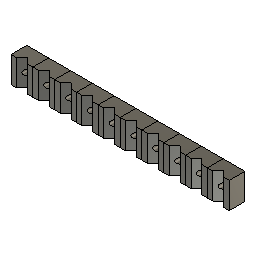
model (Autodesk Fusion 360 design; units mm, degrees)
Autodesk Fusion 360 part; units mm, degrees
sketch "profile" plane through (0, 0, 0) normal (0, 0, 1) x (1, 0, 0) in component "rail"
  line L0 (0, 0) -> (25, 0)
  line L1 (25, 0) -> (25, -18)
  line L2 (0, -18) -> (0, 0)
  line L3 (6.25, -18) -> (12.5, -11.75)
  line L4 (12.5, -11.75) -> (18.75, -18)
  line L5 (25, -18) -> (18.75, -18)
  line L6 (6.25, -18) -> (0, -18)
  line L7 (9.325, -14.925) -> (9.325, -8.575)
  line L8 (9.325, -8.575) -> (15.675, -8.575)
  line L9 (15.675, -8.575) -> (15.675, -14.925)
  line L10 (12.5, -11.75) -> (12.5, -8.575) construction
  line L11 (6.25, -18) -> (12.5, -18) construction
  line L12 (12.5, -18) -> (18.75, -18) construction
  dimension "d4" = 25
  dimension "d6" = 3.175
  dimension "d8" = 18
  dimension "d9" = 6.35
  dimension "d10" = 11.75
  constraint horizontal L0
  constraint vertical L1
  constraint horizontal L5
  constraint vertical L2
  constraint coincident L0.start L2.end
  constraint coincident L3.start L5
  constraint perpendicular L3 L4
  constraint collinear L5 L6
  constraint equal L5 L6
  constraint equal L3 L4
  constraint coincident L3 L7.start
  constraint coincident L4 L9.end
  constraint vertical L7
  constraint vertical L9
  constraint horizontal L8
  constraint midpoint L8 L10.end
  constraint vertical L10
  constraint horizontal L11
  constraint horizontal L12
  constraint equal L6 L11
  constraint equal L11 L12
  measures "d4" distance of L0.start L0.end
  measures "d6" vertical distance of L3.end L10.end
  measures "d8" distance of L0.start L2.start
  measures "d9" distance of L7 L9
  measures "d10" vertical distance of L0.end L3.end
extrude "Extrude1" add sketch "profile" along normal blind 30 makes body 1 in component "rail"
sketch "hole" plane through (0, 0, 0) normal (0, 1, 0) x (-1, 0, 0) in component "rail"
  line L0 (-25, 0) -> (0, 0)
  line L1 (0, 0) -> (0, 30)
  line L2 (0, 30) -> (-25, 30)
  line L3 (-25, 30) -> (-25, 0)
  line L4 (-25, 0) -> (0, 30) construction
  circle A0 centre (-12.5, 15) radius 3.175
  dimension "d13" = 6.35
  constraint coincident L0.start L3.end
  constraint coincident L1.end L2.start
  constraint midpoint L4 A0.centre
  measures "d13" diameter of A0
ref_plane "WorkPlane1" through (12.5, -11.75, 15) normal (0, 1, 0) x (0, 0, 1) in component "rail"
extrude "Extrude2" cut sketch "hole" along normal blind 3.175 and the other way blind 30 from surface at -11.75 contours A0 bodies 1 in component "rail"
pattern_linear "R-Pattern1" count 10 spacing 25 along (1, 0, 0) of bodies 1 makes body 2 at (33.3333, 0, 20) makes body 3 at (58.3333, 0, 20) makes body 4 at (83.3333, 0, 20) makes body 5 at (108.3333, 0, 20) makes body 6 at (133.3333, 0, 20) makes body 7 at (158.3333, 0, 20) makes body 8 at (183.3333, 0, 20) makes body 9 at (208.3333, 0, 20) makes body 10 at (233.3333, 0, 20) in component "rail"
component "rail" placed x (1, 0, 0) y (0, 1, 0) z (0, 0, 1) at (0, 0, 0)
equation "spacing = 25 mm"
equation "height = 30 mm"
equation "magDiameter = 1/4\""
equation "d4 = spacing"
equation "magDepth = 1/8\""
equation "d6 = magDepth"
equation "d9 = magDiameter"
equation "d11 = height"
equation "d13 = magDiameter"
equation "d16 = magDepth"
equation "d22 = spacing"
